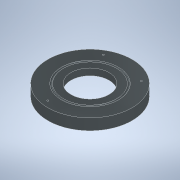
# Autodesk Inventor part: Корпус дросселя
Saved by Autodesk Inventor 2021 (Build 250183000, 183)
## iProperties
Created: 2020-11-05
Part Number: Корпус дросселя
Material: Чугун, серый
Document SubType Name: Modeling
Designer: Тимоха
Density: 7.15 g/cm^3
Appearance: Чугун серый
Mass: 1127.79 g
Surface Area: 355.126 cm^2
Volume: 157.733 cm^3
Author: Тимоха
Autodesk Inventor part; units mm, degrees
ref_plane "YZ Plane" through (0, 0, 0) normal (1, 0, 0) x (0, 1, 0)
ref_plane "XZ Plane" through (0, 0, 0) normal (0, 1, 0) x (-1, 0, 0)
ref_plane "XY Plane" through (0, 0, 0) normal (0, 0, 1) x (1, 0, 0)
sketch "Эскиз1" plane through (0, 0, 0) normal (0, 0, 1) x (1, 0, 0)
  line L0 (0, 0) -> (0, 8)
  line L1 (0, 8) -> (0, 16)
  line L2 (0, 0) -> (0, 20)
  line L3 (0, 20) -> (-75, 20)
  line L4 (-75, 20) -> (-75, 0)
  line L5 (-75, 0) -> (-51, 0)
  line L6 (-51, 0) -> (-51, 8)
  line L7 (-51, 8) -> (-34, 8)
  line L8 (-34, 8) -> (-34, 20)
  line L9 (0, 20) -> (-49, 20)
  line L10 (-49, 20) -> (-49, 20)
  circle A0 centre (-49, 20) radius 2
  point P0 (-47, 20)
  point P1 (-51, 20)
  dimension "d22" = 20
  dimension "d23" = 75
  dimension "d26" = 24
  dimension "d27" = 8
  dimension "d28" = 17
  dimension "d29" = 49
  dimension "d30" = 0
  dimension "d31" = 4
  constraints: 22 end point, 5 perpendicular, 3 point on line, 3 vertical, 1 centre point, 1 coincident, 1 horizontal
  measures "d22" distance of L0.start L2.end
  measures "d23" distance of L2.end L3.end
  measures "d26" distance of L4.end L5.end
  measures "d27" distance of L5.end L6.end
  measures "d28" distance of L6.end L7.end
  measures "d29" distance of L2.end L9.end
  measures "d30" distance of L9.end L10.end
  measures "d31" diameter of A0
revolve "Вращение1" add sketch "Эскиз1" angle 360 about axis through (0, 8, 0) along (0, 1, 0) contours L8 L7 L6 L5 L4 L3 A0
sketch "Эскиз2" plane through (0, 20, 0) normal (0, 1, 0) x (1, 0, 0)
  line L0 (0, 0) -> (41.7812, 49.7929)
  line L1 (0, 0) -> (65, 0) construction
  line L2 (0, 0) -> (-32.5, 56.2917)
  line L3 (0, 0) -> (65, 0) construction
  line L4 (0, 0) -> (-11.2871, -64.0125)
  line L5 (0, 0) -> (65, 0) construction
  circle A0 centre (-32.5, 56.2917) radius 1.5
  circle A1 centre (41.7812, 49.7929) radius 1.5
  circle A2 centre (-11.2871, -64.0125) radius 1.5
  dimension "d11" = 65
  dimension "d12" = 50
  dimension "d13" = 65
  dimension "d14" = 120
  dimension "d15" = 65
  dimension "d16" = 100
  dimension "d17" = 3
  dimension "d18" = 3
  dimension "d19" = 3
  constraints: 12 end point, 3 centre point, 3 coincident, 3 equal length, 3 horizontal
  measures "d11" distance of L0.start L0.end
  measures "d12" angle of L1 L0
  measures "d13" distance of L0.start L2.end
  measures "d14" angle of L3 L2
  measures "d15" distance of L0.start L4.end
  measures "d16" angle of L4 L5
  measures "d17" diameter of A0
  measures "d18" diameter of A1
  measures "d19" diameter of A2
extrude "Выдавливание1" cut sketch "Эскиз2" against normal through all
sketch "Эскиз3" plane through (0, 0, 0) normal (0, -1, 0) x (1, 0, 0)
  circle A0 centre (0, 0) radius 53
  circle A1 centre (0, 0) radius 55
  dimension "d32" = 106
  dimension "d33" = 110
  constraints: 2 centre point, 2 coincident
  measures "d32" diameter of A0
  measures "d33" diameter of A1
extrude "Выдавливание2" cut sketch "Эскиз3" against normal blind 1.5
